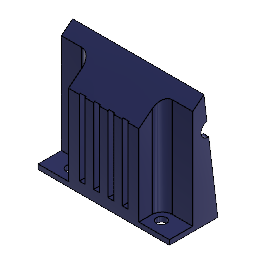
1-hotend_wire_cover_V3 v2 (Autodesk Fusion 360 design; units mm, degrees)
Autodesk Fusion 360 part; units mm, degrees
sketch "MainProfile" plane through (0, 0, 0) normal (0, 0, 1) x (1, 0, 0)
  line L0 (-23, 0) -> (23, 0)
  line L1 (23, 0) -> (23, -17)
  line L2 (23, -17) -> (-23, -17)
  line L3 (-23, -17) -> (-23, 0)
  line L4 (-23, -17) -> (-12.3, -17)
  line L5 (-12.3, -17) -> (-12.3, -8.85)
  line L6 (-12.3, -8.85) -> (-23, -8.85)
  line L7 (-23, -8.85) -> (-23, -17)
  circle A0 centre (-15.77, -12.57) radius 1.75
  line L8 (0, 0) -> (0, -17) construction
  line L9 (12.3, -8.85) -> (23, -8.85)
  line L10 (12.3, -17) -> (12.3, -8.85)
  circle A1 centre (15.77, -12.57) radius 1.75
  line L11 (-17, 0) -> (-17, -4.3)
  line L12 (-17, -4.3) -> (17, -4.3)
  line L13 (17, -4.3) -> (17, 0)
  arc A2 (-9.8976, -4.3) -> (9.8976, -4.3) centre (0, -4.52) ccw
  dimension "d1" = 46
  dimension "d2" = 17
  dimension "d3" = 10.7
  dimension "d4" = 8.15
  dimension "d5" = 3.5
  dimension "d6" = 4.43
  dimension "d7" = 7.23
  dimension "d8" = 6
  dimension "d9" = 6
  dimension "d10" = 4.3
  dimension "d11" = 9.9
  dimension "d12" = 4.52
  constraint horizontal L0
  constraint vertical L1
  constraint horizontal L2
  constraint vertical L3
  constraint midpoint L8.start L0
  constraint horizontal L4
  constraint vertical L5
  constraint horizontal L6
  constraint vertical L7
  constraint coincident L8.start origin
  constraint midpoint L2 L8.end
  constraint symmetric L4.end L8 L10.start
  constraint symmetric L5.end L8 L9.start
  constraint symmetric L6.end L8 L9.end
  constraint symmetric A0 L8 A1
  constraint coincident L0 L11.start
  constraint perpendicular L0 L11
  constraint perpendicular L11 L12
  constraint coincident L0 L13.end
  constraint perpendicular L0 L13
  constraint coincident L12 A2.end
  constraint coincident L12 A2.start
  constraint vertical L8.start A2.centre
  measures "d1" distance of L1 L3
  measures "d2" distance of L0 L2
  measures "d3" distance of L2.end L4.end
  measures "d4" distance of L2.end L6.end
  measures "d5" diameter of A0
  measures "d6" distance of L4 A0.centre
  measures "d7" distance of L3 A0.centre
  measures "d8" distance of L1 L13
  measures "d9" distance of L3 L11
  measures "d10" distance of L0 L12
  measures "d11" radius of A2
  measures "d12" distance of L8.start A2.centre
extrude "Extrude1" add sketch "MainProfile" along normal blind 40 contours L0 L1 L2 L3 L5 L6 L9 L10 L11 L12 L13 A2 | L0 L11 L12 L13 | L12 A2
fillet "Fillet1" radius 3.5 2 edges at (12.3, -8.85, 20) (-12.3, -8.85, 20)
chamfer "Chamfer1" distance 12.5 distance2 10 1 edges at (0, -17, 40) measured on face at (-4.6359, -3.1352, 40)
draft "Draft1" angle -7 neutral plane through (0, 0, 0) pull (0, 0, -1) 1 faces at (-7.6667, 0, 13.3333)
shell "Shell1" thickness 2 removed faces 1 at (7.6667, -1.6249, 13.2334)
extrude "Extrude2" cut sketch "MainProfile" along normal blind 3.514 contours L0 L11 L12 L13 | L12 A2
extrude "Extrude3" add sketch "MainProfile" along normal blind 1.75 contours L2 L3 L4 L5 L6 L7 | L1 L2 L9 L10
sketch "Slots" plane through (0, 0, 0) normal (0, 1, 0) x (1, 0, 0)
  line L0 (8.5, -3.75) -> (6.5, -3.75)
  line L1 (6.5, -3.75) -> (6.5, -30.25)
  line L2 (6.5, -30.25) -> (8.5, -30.25)
  line L3 (8.5, -30.25) -> (8.5, -3.75)
  line L4 (3.5, -3.75) -> (1.5, -3.75)
  line L5 (1.5, -3.75) -> (1.5, -30.25)
  line L6 (3.5, -30.25) -> (3.5, -3.75)
  line L7 (1.5, -30.25) -> (3.5, -30.25)
  line L8 (-1.5, -3.75) -> (-3.5, -3.75)
  line L9 (-3.5, -3.75) -> (-3.5, -30.25)
  line L10 (-1.5, -30.25) -> (-1.5, -3.75)
  line L11 (-3.5, -30.25) -> (-1.5, -30.25)
  line L12 (-6.5, -3.75) -> (-8.5, -3.75)
  line L13 (-8.5, -3.75) -> (-8.5, -30.25)
  line L14 (-6.5, -30.25) -> (-6.5, -3.75)
  line L15 (-8.5, -30.25) -> (-6.5, -30.25)
  dimension "d25" = 2
  dimension "d26" = 26.5
  dimension "d27" = 6.5
  dimension "d28" = 3.75
  dimension "d31" = -5
  dimension "d32" = 0
  constraint horizontal L0
  constraint vertical L1
  constraint horizontal L2
  constraint vertical L3
  measures "d25" distance of L1 L3
  measures "d26" distance of L0 L2
  measures "d27" distance of origin L1
  measures "d28" distance of origin L0
extrude "Extrude4" cut sketch "Slots" against normal blind 24.407
sketch "Side" plane through (0, 0, 0) normal (1, 0, 0) x (0, 1, 0)
  circle A0 centre (-0.3374, 8.2763) radius 2.75
  circle A1 centre (-3.438, 28.558) radius 2.5
  dimension "d35" = 5.5
  dimension "d36" = 5
  dimension "d37" = 0.3374
  dimension "d38" = 8.2763
  dimension "d39" = 28.558
  dimension "d40" = 3.438
  measures "d35" diameter of A0
  measures "d36" diameter of A1
  measures "d37" horizontal distance of origin A0.centre
  measures "d38" vertical distance of origin A0.centre
  measures "d39" vertical distance of origin A1.centre
  measures "d40" horizontal distance of origin A1.centre
extrude "Extrude5" cut sketch "Side" along normal blind 28.202 contours A1
extrude "Extrude6" cut sketch "Side" against normal blind 29.648 contours A0
